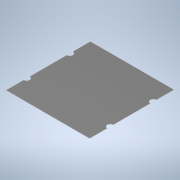
# Autodesk Inventor part: Coverplate Film
Saved by Autodesk Inventor 2022 (Build 260153000, 153)
## iProperties
Created: 2022-02-23
Part Number: Coverplate Film
Material: Thermoplastic Resin
Document SubType Name: Modeling
Designer: Caleb
Density: 1.28 g/cm^3
Appearance: Smooth - Black
Author: Caleb
Autodesk Inventor part; units mm, degrees
ref_plane "YZ Plane" through (0, 0, 0) normal (1, 0, 0) x (0, 1, 0)
ref_plane "XZ Plane" through (0, 0, 0) normal (0, 1, 0) x (-1, 0, 0)
ref_plane "XY Plane" through (0, 0, 0) normal (0, 0, 1) x (1, 0, 0)
sketch "Sketch1" plane through (0, 0, 0) normal (0, 1, 0) x (-1, 0, 0)
  line L0 (-20.8, -21) -> (20.8, -21)
  line L1 (20.8, -21) -> (20.8, 21)
  line L2 (20.8, 21) -> (-20.8, 21)
  line L3 (-20.8, 21) -> (-20.8, -21)
  line L4 (-20.8, -21) -> (20.8, 21) construction
  line L5 (20.8, -21) -> (-20.8, 21) construction
  point P0 (0, 0)
  dimension "d0" = 42
  dimension "d1" = 41.6
  constraints: 12 end point, 2 midpoint, 2 parallel, 1 horizontal, 1 perpendicular
  measures "d0" distance of L0.end L1.end
  measures "d1" distance of L1.end L2.end
extrude "Extrusion1" add sketch "Sketch1" along normal blind 0.08
sketch "Sketch2" plane through (0, 0.08, 0) normal (0, 1, 0) x (1, 0, 0)
  arc A0 (-20.8, 9.225) -> (-20.8, 12.225) centre (-20.8, 10.725) ccw
  line L0 (0, -4.1299) -> (0, 4.8188) construction
  arc A1 (20.8, 12.225) -> (20.8, 9.225) centre (20.8, 10.725) ccw
  line L1 (20.8, -21) -> (20.8, 21) projected
  line L2 (-20.8, 21) -> (-20.8, -21) projected
  line L3 (20.8, 21) -> (-20.8, 21) projected
  line L4 (-26.5331, 0) -> (30.3712, 0)
  arc A2 (-20.8, -12.225) -> (-20.8, -9.225) centre (-20.8, -10.725) ccw
  arc A3 (20.8, -9.225) -> (20.8, -12.225) centre (20.8, -10.725) ccw
  point P0 (0, 0)
  point P1 (20.8, -9.225)
  point P2 (20.8, -12.225)
  point P3 (-20.8, 9.225)
  point P4 (-20.8, -12.225)
  point P5 (-20.8, -9.225)
  dimension "d5" = 1.5
  dimension "d8" = 3
  dimension "d9" = 10.275
  constraints: 9 symmetric about line, 8 point on circle, 4 centre point, 4 end point, 1 horizontal, 1 point on line, 1 vertical, 3 other
  measures "d5" radius of A0
  measures "d8" distance of A0.start A0.end
  measures "d9" distance from line of L3 A0.centre
extrude "Extrusion2" cut sketch "Sketch2" against normal through all contours L2 A0 | A1 L1 | A3 L1 | A2 L2
body "Solid1"
